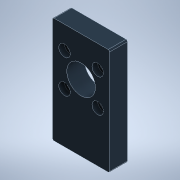
# Autodesk Inventor part: Soporte1_CilindroHorizontal
Saved by Autodesk Inventor 2021 (Build 250183000, 183)
## iProperties
Created: 2021-07-10
Part Number: Soporte1_CilindroHorizontal
Material: Generic
Document SubType Name: Modeling
Designer: Nelson
Density: 1 g/cm^3
Appearance: Default(1)
Author: Nelson
Autodesk Inventor part; units mm, degrees
ref_plane "YZ Plane" through (0, 0, 0) normal (1, 0, 0) x (0, 1, 0)
ref_plane "XZ Plane" through (0, 0, 0) normal (0, 1, 0) x (-1, 0, 0)
ref_plane "XY Plane" through (0, 0, 0) normal (0, 0, 1) x (1, 0, 0)
sketch "Sketch1" plane through (0, 0, 0) normal (0, 0, 1) x (1, 0, 0)
  line L0 (0, 0) -> (80, 0)
  line L1 (80, 0) -> (80, 148.736)
  line L2 (80, 148.736) -> (0, 148.736)
  line L3 (0, 148.736) -> (0, 0)
  circle A0 centre (40, 93.486) radius 20
  circle A1 centre (16.75, 116.736) radius 4.5
  circle A2 centre (63.25, 116.736) radius 4.5
  circle A3 centre (16.75, 70.236) radius 4.5
  circle A4 centre (63.25, 70.236) radius 4.5
  dimension "d0" = 40
  dimension "d1" = 23.25
  dimension "d2" = 23.25
  dimension "d3" = 23.25
  dimension "d4" = 23.25
  dimension "d5" = 23.25
  dimension "d6" = 23.25
  dimension "d7" = 23.25
  dimension "d8" = 23.25
  dimension "d9" = 9
  dimension "d10" = 93.486
  dimension "d11" = 80
  dimension "d12" = 40
  dimension "d13" = 32
  constraints: 8 end point, 5 centre point, 3 equal radius, 2 parallel, 1 horizontal, 1 perpendicular
  measures "d0" diameter of A0
  measures "d1" horizontal distance of A0.centre A1.centre
  measures "d2" horizontal distance of A0.centre A1.centre
  measures "d3" horizontal distance of A2.centre A0.centre
  measures "d4" horizontal distance of A0.centre A2.centre
  measures "d5" horizontal distance of A3.centre A0.centre
  measures "d6" horizontal distance of A3.centre A0.centre
  measures "d7" horizontal distance of A4.centre A0.centre
  measures "d8" horizontal distance of A0.centre A4.centre
  measures "d9" diameter of A1
  measures "d10" distance from line of L0 A0.centre
  measures "d11" distance of L0.start L0.end
  measures "d12" distance from line of L3 A0.centre
  measures "d13" distance from line of L2 A1.centre
extrude "Extrusion1" add sketch "Sketch1" against normal blind 25
sketch "Sketch2" plane through (0, 0, 0) normal (0, 0, 1) x (1, 0, 0)
  circle A0 centre (16.75, 116.736) radius 4.5 projected
  circle A1 centre (63.25, 116.736) radius 4.5 projected
  circle A2 centre (16.75, 70.236) radius 4.5 projected
  circle A3 centre (63.25, 70.236) radius 4.5 projected
  circle A4 centre (16.75, 116.736) radius 8
  circle A5 centre (63.25, 116.736) radius 8
  circle A6 centre (16.75, 70.236) radius 8
  circle A7 centre (63.25, 70.236) radius 8
  point P0 (0, 0)
  dimension "d16" = 16
  dimension "d17" = 16
  dimension "d18" = 16
  dimension "d19" = 16
  constraints: 4 centre point, 4 coincident
  measures "d16" diameter of A4
  measures "d17" diameter of A5
  measures "d18" diameter of A6
  measures "d19" diameter of A7
extrude "Extrusion2" cut sketch "Sketch2" against normal blind 8 contours A0 | A1 | A2 | A3 | A4 | A5 | A6 | A7
fillet "Fillet1" radius 2 4 edges at (80, 148.736, -12.5) (0, 148.736, -12.5) (80, 0, -12.5) (0, 0, -12.5)
sketch "Sketch3" plane through (2, 0, 0) normal (0, -1, 0) x (1, 0, 0)
  line L0 (-2, 0) -> (-2, -25) projected
  line L1 (78, -25) -> (78, 0) projected
  line L2 (0, 0) -> (76, 0) projected
  point P0 (20, -12.5)
  point P1 (56, -12.5)
  dimension "d28" = 22
  dimension "d29" = 12.5
  dimension "d30" = 22
  dimension "d31" = 12.5
  measures "d28" distance from line of point (20, -12.5) L0
  measures "d29" distance from line of L2 point (20, -12.5)
  measures "d30" distance from line of L1 point (56, -12.5)
  measures "d31" distance from line of L2 point (56, -12.5)
hole "Hole1" at (58, 0, -12.5) at (22, 0, -12.5) direction (0, 1, 0) diameter 8.376 depth 25 tip angle 137 thread size "M10x1.5" class "6H" standard "ISO Metric profile"
equation "\"d2\" = d1"
equation "\"d3\" = d1"
equation "\"d4\" = d1"
equation "\"d5\" = d1"
equation "\"d6\" = d1"
equation "\"d7\" = d1"
equation "\"d8\" = d1"
equation "\"d12\" = 0.5 * d11"
equation "\"d30\" = d28"
equation "\"d31\" = d29"
body "Solid1"
